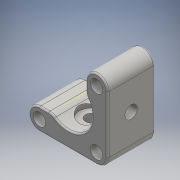
# Autodesk Inventor part: polaris_K05_main
Saved by Autodesk Inventor 2016 (Build 200138000, 138)
## iProperties
Created: 2015-09-04
Part Number: polaris_K05_main
Material: Generic
Document SubType Name: Modeling
Designer: HE BEC
Density: 1 g/cm^3
Appearance: Default
Author: HE BEC
Autodesk Inventor part; units mm, degrees
ref_plane "YZ Plane" through (0, 0, 0) normal (1, 0, 0) x (0, 1, 0)
ref_plane "XZ Plane" through (0, 0, 0) normal (0, 1, 0) x (-1, 0, 0)
ref_plane "XY Plane" through (0, 0, 0) normal (0, 0, 1) x (1, 0, 0)
sketch "Sketch1" plane through (0, 0, 0) normal (0, 1, 0) x (-1, 0, 0)
  line L0 (0, 0) -> (25.4, 0)
  line L1 (25.4, 0) -> (25.4, 25.4)
  line L2 (25.4, 25.4) -> (0, 25.4)
  line L3 (0, 25.4) -> (0, 0)
  circle A0 centre (3.5, 21.9) radius 2
  circle A1 centre (21.9, 3.5) radius 2
  circle A2 centre (12.7, 12.7) radius 7.625
  circle A3 centre (3.5, 3.5) radius 2
  dimension "d1" = 25.4
  dimension "d2" = 12.7
  dimension "d3" = 12.7
  dimension "d4" = 3.5
  dimension "d5" = 3.5
  dimension "d6" = 3.5
  dimension "d7" = 3.5
  dimension "d11" = 4
  dimension "d12" = 15.25
  constraints: 8 end point, 4 centre point, 4 coincident, 2 equal radius, 2 parallel, 2 perpendicular, 1 horizontal, 1 horizontal alignment, 1 vertical alignment
  measures "d1" distance of L0.end L1.end
  measures "d2" distance from line of L0 point (12.7, 12.7)
  measures "d3" distance from line of L3 point (12.7, 12.7)
  measures "d4" distance from line of L3 point (3.5, 21.9)
  measures "d5" distance from line of L2 point (3.5, 21.9)
  measures "d6" distance from line of L0 point (21.9, 3.5)
  measures "d7" distance from line of L1 point (21.9, 3.5)
  measures "d11" diameter of A1
  measures "d12" diameter of A2
extrude "Extrusion1" add sketch "Sketch1" along normal blind 15.2
sketch "Sketch3" plane through (0, 0, 0) normal (0, -1, 0) x (1, 0, 0)
  line L0 (-25.4, 0) -> (-25.4, 25.4) projected
  line L1 (-25.4, 25.4) -> (-7, 25.4)
  line L2 (-7, 25.4) -> (-7, 7.6354)
  line L3 (-7.6354, 7) -> (-25.4, 7)
  line L4 (-25.4, 7) -> (-25.4, 25.4)
  line L5 (0, 25.4) -> (0, 0) projected
  line L6 (0, 0) -> (-25.4, 0) projected
  circle A0 centre (-12.7, 12.7) radius 7.625 projected
  arc A1 (-7.6354, 7) -> (-7, 7.6354) centre (-12.7, 12.7) ccw
  dimension "d13" = 7
  constraints: 8 end point, 2 parallel, 2 point on circle, 1 centre point, 1 coincident, 1 horizontal, 1 perpendicular, 2 other
  measures "d13" distance between parallel lines of L5 L2
extrude "Extrusion2" cut sketch "Sketch3" against normal through all contours L0 L1 L2 A0 L3 | A0 L2 L3
fillet "Fillet1" radius 3.5 7 edges at (-7, 7.6, 17.7646) (-7, 7.6, 25.4) (0, 7.6, 25.4) (0, 7.6, 0) (-17.7646, 7.6, 7) (-25.4, 7.6, 7) (-25.4, 7.6, 0)
sketch "Sketch4" plane through (-3.5, 0, 0) normal (0, 0, -1) x (-1, 0, 0)
  circle A0 centre (9.2, 7.6) radius 2
  line L0 (0, 15.2) -> (18.4, 15.2) projected
  line L1 (-3.5, 15.2) -> (-3.5, 0) projected
  line L2 (-3.5, 15.2) -> (0, 15.2) projected
  dimension "d18" = 4
  dimension "d20" = 12.7
  dimension "d32" = 7.6
  dimension "d33" = 15.2
  constraints: 1 centre point
  measures "d18" diameter of A0
  measures "d20" distance from line of L1 A0.centre
  measures "d32" distance from line of L2 A0.centre
  measures "d33" distance of L1.start L1.end
extrude "Extrusion3" cut sketch "Sketch4" against normal through all
ref_plane "Work Plane1" through (-3.5, 0, 4.6) normal (0, 0, -1) x (-1, 0, 0)
sketch "Sketch5" plane through (-3.5, 0, 4.6) normal (0, 0, -1) x (-1, 0, 0)
  circle A0 centre (9.2, 7.6) radius 4
  circle A1 centre (9.2, 7.6) radius 2 projected
  point P0 (-3.5, 0)
  dimension "d26" = 8
  constraints: 1 centre point, 1 concentric
  measures "d26" diameter of A0
extrude "Extrusion4" cut sketch "Sketch5" against normal through all
fillet "Fillet2" radius 0.5 1 edges at (-7.3083, 0, 7.3083)
fillet "Fillet3" radius 0.5 1 edges at (-7.3083, 15.2, 7.3083)
pattern_circular "Circular Pattern1" count 2 over 90 about axis through (-12.7, 0, 12.7) along (0, -1, 0) of "Extrusion4", "Extrusion3"
equation "\"d2\" = 0.5 * d1"
equation "\"d3\" = d2"
equation "\"d5\" = d4"
equation "\"d6\" = d7"
equation "\"d7\" = d5"
equation "\"d13\" = 2 * d4"
equation "\"d20\" = 0.5 * d1"
equation "\"d32\" = 0.5 * d33"
body "Solid1"
